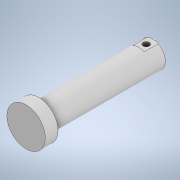
# Autodesk Inventor part: Trzemień
Saved by Autodesk Inventor 2022 (Build 260153000, 153)
## iProperties
Created: 2024-01-14
Part Number: Trzemień
Material: Generic
Document SubType Name: Modeling
Designer: mateu
Density: 1 g/cm^3
Appearance: Default
Author: mateu
Autodesk Inventor part; units mm, degrees
ref_plane "YZ Plane" through (0, 0, 0) normal (1, 0, 0) x (0, 1, 0)
ref_plane "XZ Plane" through (0, 0, 0) normal (0, 1, 0) x (-1, 0, 0)
ref_plane "XY Plane" through (0, 0, 0) normal (0, 0, 1) x (1, 0, 0)
sketch "Sketch1" plane through (0, 0, 0) normal (0, 0, 1) x (1, 0, 0)
  circle A0 centre (0, 0) radius 7.5
  constraints: 1 centre point, 1 coincident
extrude "Extrusion1" add sketch "Sketch1" along normal blind 5
sketch "Sketch2" plane through (0, 0, 0) normal (0, 0, -1) x (-1, 0, 0)
  circle A0 centre (0, 0) radius 5
  constraints: 1 centre point, 1 coincident
extrude "Extrusion2" add sketch "Sketch2" along normal blind 45
fillet "Fillet1" radius 0.5 1 edges at (5, 0, -45)
sketch "Sketch3" plane through (0, 0, -45) normal (0, 0, -1) x (-1, 0, 0)
  point P0 (0, 0)
sketch "Sketch4" plane through (0, 0, -45) normal (0, 0, -1) x (-1, 0, 0)
  line L0 (0, 4.5) -> (5, 4.5)
  line L1 (5, 4.5) -> (5, 5.5)
  line L2 (5, 5.5) -> (-5, 5.5)
  line L3 (-5, 5.5) -> (-5, 4.5)
  line L4 (-5, 4.5) -> (0, 4.5)
  circle A0 centre (0, 0) radius 4.5 projected
  constraints: 10 end point, 2 perpendicular, 1 horizontal, 1 point on line, 1 tangent
extrude "Extrusion3" cut sketch "Sketch4" against normal blind 6 contours L4 L3 L2 L1 L0
sketch "Sketch5" plane through (-2.1794, 4.5, -39) normal (0, 1, 0) x (1, 0, 0)
  point P0 (2.1794, -39)
  point P1 (2.1794, 6)
sketch "Sketch6" plane through (-2.1794, 4.5, -39) normal (0, 1, 0) x (1, 0, 0)
  point P0 (2.1794, -39)
sketch "Sketch7" plane through (-2.1794, 4.5, -39) normal (0, 1, 0) x (1, 0, 0)
  point P0 (2.1794, -39)
sketch "Sketch8" plane through (-2.1794, 4.5, -39) normal (0, 1, 0) x (1, 0, 0)
  point P0 (2.1794, -39)
  point P1 (2.1794, -3)
  point P2 (2.1794, -3)
  point P3 (2.1794, 3)
  constraints: 1 coincident
hole "Hole1" at (0, 4.5, -42) direction (0, -1, 0) diameter 2.459 depth 8.8 tip angle 118 thread size "M3x0.5" class "6H" standard "ISO Metric profile"
body "Solid1"
